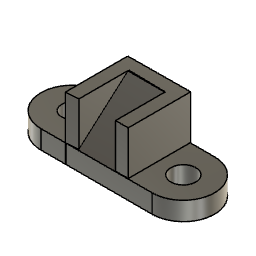
A2 (Autodesk Fusion 360 design; units mm, degrees)
Autodesk Fusion 360 part; units mm, degrees
sketch "Base" plane through (0, 0, 0) normal (0, 0, 1) x (1, 0, 0)
  line L0 (57, 32) -> (-57, 32)
  line L1 (-57, -32) -> (57, -32)
  circle A0 centre (-57, 0) radius 11
  circle A1 centre (57, 0) radius 12.8062
  line L2 (57, 32) -> (57, -32) construction
  line L3 (-57, 32) -> (-57, -32) construction
  arc A2 (-57, 32) -> (-57, -32) centre (-57, 0) ccw
  arc A3 (57, -32) -> (57, 32) centre (57, 0) ccw
  dimension "d1" = 114
  dimension "d2" = 64
  dimension "d3" = 22
  dimension "d4" = 25.6125
  constraint horizontal L0
  constraint parallel L0 L1
  constraint concentric A0 A2
  constraint concentric A1 A3
  constraint perpendicular L1 L2
  constraint perpendicular L1 L3
  measures "d1" distance of L1.start L1.end
  measures "d2" distance of L0.end L1.start
  measures "d3" diameter of A0
  measures "d4" diameter of A1
extrude "Extrude1" add sketch "Base" along normal blind 19 makes body 1
sketch "Walls" plane through (0, 0, 0) normal (0, 0, 1) x (1, 0, 0)
  line L0 (-32, 31.9499) -> (-32, -32.0501)
  line L1 (32, 32.507) -> (32, -31.493)
  line L2 (-19, 20) -> (-19, -31)
  line L3 (57, 32) -> (57, -32)
  line L4 (19, -31.6163) -> (19, 19.3837)
  line L5 (-32, 31.9499) -> (32, 32.507)
  line L6 (-19, 20) -> (19, 19.3837)
  line L7 (-32, -32.0501) -> (-19, -31)
  line L8 (19, -31.6163) -> (32, -31.493)
  dimension "d7" = 64
  dimension "d9" = 64
  dimension "d10" = 51
  dimension "d12" = 25
  dimension "d15" = 51
  dimension "d16" = 51
  dimension "d17" = 13
  dimension "d18" = 51
  dimension "d19" = 13
  constraint vertical L0
  constraint vertical L1
  constraint vertical L2
  constraint vertical L4
  measures "d7" distance of L0.start L0.end
  measures "d9" distance of L1.start L1.end
  measures "d10" distance of L2.start L2.end
  measures "d12" distance of L1 L3
  measures "d15" distance of L2.start L2.end
  measures "d16" distance of L2.start L2.end
  measures "d17" distance of L0 L2
  measures "d18" distance of L4.start L4.end
  measures "d19" distance of L1 L4
extrude "Extrude3" add sketch "Walls" along normal blind 64 bodies 1
sketch "Sketch6" plane through (0, 0, 0) normal (0, 1, 0) x (1, 0, 0)
  line L0 (0, 0) -> (51, 0)
  line L1 (0, 0) -> (0, -45)
  line L2 (0, -45) -> (51, 0)
  dimension "d24" = 51
  dimension "d25" = 45
  constraint coincident L0.start L1.start
  constraint horizontal L0
  constraint perpendicular L0 L1
  measures "d24" distance of L0.start L0.end
  measures "d25" distance of L0.start L1.end
extrude "Extrude4" add sketch "Sketch6" along normal mid plane 38 separate body makes body 2
move_body "Move1" bodies 2 to x (0, -1, 0) y (1, 0, 0) z (0, 0, 1) at (10.5264, 7.3398, 34.8134)
move_body "Move2" bodies 2 to x (1, 0, 0) y (0, 1, 0) z (0, 0, 1) at (11.6573, -15.4638, 12.2492)
move_body "Move3" bodies 2 to x (1, 0, 0) y (0, 1, 0) z (0, 0, 1) at (-22.4988, 27.4496, -28.445)
named bodies: "Base"
